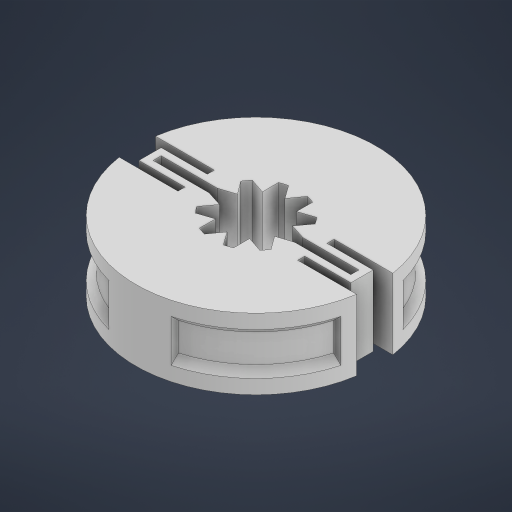
# Autodesk Inventor part: gear_grip
Saved by Autodesk Inventor 2024 (Build 280153000, 153)
## iProperties
Created: 2024-10-06
Part Number: gear_grip
Material: Generic
Document SubType Name: Modeling
Designer: loren
Density: 1 g/cm^3
Appearance: Default
Author: loren
## iProperties of the stored document gear-grip_3DPrint.ipt
Created: 2026-02-06
Part Number: gear-grip_3DPrint
Material: Generic
Document SubType Name: Modeling
Designer: lokies
Density: 1 g/cm^3
Appearance: Default
Author: lokies
Autodesk Inventor part; units mm, degrees
ref_plane "YZ Plane" through (0, 0, 0) normal (1, 0, 0) x (0, 1, 0)
ref_plane "XZ Plane" through (0, 0, 0) normal (0, 1, 0) x (-1, 0, 0)
ref_plane "XY Plane" through (0, 0, 0) normal (0, 0, 1) x (1, 0, 0)
sketch "Sketch1" plane through (0, 0, 0) normal (0, 0, 1) x (1, 0, 0)
  circle A0 centre (0, 0) radius 8.5
  dimension "d0" = 17
  constraints: 1 centre point, 1 coincident
  measures "d0" diameter of A0
extrude "Extrusion1" add sketch "Sketch1" along normal mid plane 5
sketch "Sketch2" plane through (0, 0, 2.5) normal (0, 0, 1) x (1, 0, 0)
  circle A0 centre (0, 0) radius 3.05
  dimension "d3" = 6.1
  constraints: 1 centre point, 1 coincident
  measures "d3" diameter of A0
extrude "Extrusion2" cut sketch "Sketch2" against normal through all
sketch "Sketch3" plane through (0, 0, 2.5) normal (0, 0, 1) x (1, 0, 0)
  circle A0 centre (0, 0) radius 3.05
  line L0 (-0.665337, 2.976546) -> (0, 2.05)
  line L1 (0, 2.05) -> (0.665337, 2.976546)
  line L2 (0, 2.05) -> (0, 3.05) construction
  dimension "d6" = 25.2
  dimension "d7" = 1
  constraints: 6 end point, 3 point on circle, 1 equal length, 1 horizontal alignment, 1 vertical
  measures "d7" distance of L0.end L2.end
extrude "Extrusion3" add sketch "Sketch3" against normal up to surface (5 mm away) contours L1 L0 A0 picked at (0.296238, 2.689452)
pattern_circular "Circular Pattern1" count 10 over 360 about axis through (0, 0, -10) along (0, 0, 1) of "Extrusion3"
chamfer "Chamfer1" distance 0.5 angle 45 33 edges at (-0.3327, -2.5133, -2.5) (0.3327, -2.5133, -2.5) (0.9425, -2.9007, -2.5) (-0.9425, -2.9007, -2.5) (1.2081, -2.2288, -2.5) (2.4675, -1.7927, -2.5) (1.7464, -1.8377, -2.5) (2.2875, -1.093, -2.5) (2.4931, 0.4603, -2.5) (2.2875, 1.093, -2.5) (2.4675, 1.7927, -2.5) (1.7464, 1.8377, -2.5) (1.2081, 2.2288, -2.5) (0.9425, 2.9007, -2.5) (0.3327, 2.5133, -2.5) (-0.3327, 2.5133, -2.5) (-0.9425, 2.9007, -2.5) (-1.2081, 2.2288, -2.5) (-1.7464, 1.8377, -2.5) (-2.4675, 1.7927, -2.5) (-2.2875, 1.093, -2.5) (-2.4931, 0.4603, -2.5) (-3.05, 0, -2.5) (-2.4931, -0.4603, -2.5) (-2.2875, -1.093, -2.5) (-2.4675, -1.7927, -2.5) (-1.7464, -1.8377, -2.5) (-1.2081, -2.2288, -2.5) (2.4931, -0.4603, -2.5) (3.0466, 0.1437, -2.5) (2.9007, 0.9425, -2.5) (2.9007, -0.9425, -2.5) (3.0466, -0.1437, -2.5)
sketch "Sketch5" plane through (0, 0, 2.5) normal (0, 0, 1) x (1, 0, 0)
  arc A0 (3.036464, -0.28703) -> (3.036464, 0.28703) centre (0, 0) ccw
  line L0 (3.036464, 0.28703) -> (7, 0.28703)
  line L1 (7, 0.28703) -> (7, -0.28703)
  line L2 (7, -0.28703) -> (3.036464, -0.28703)
  line L3 (3.036464, -0.28703) -> (3.036464, 0.28703)
  circle A1 centre (0, 0) radius 8.5
  line L4 (7.5, 0.78703) -> (4.236464, 0.78703)
  line L5 (4.236464, 0.78703) -> (4.236464, 1.28703)
  line L6 (4.236464, 1.28703) -> (8.401997, 1.28703)
  line L7 (7.5, -0.78703) -> (4.236464, -0.78703)
  line L8 (4.236464, -0.78703) -> (4.236464, -1.28703)
  line L9 (4.236464, -1.28703) -> (8.401997, -1.28703)
  line L10 (7.5, 0.78703) -> (7.5, -0.78703)
  point P0 (8.401997, -1.28703)
  point P1 (8.401997, 1.28703)
  dimension "d19" = 0.5
  dimension "d20" = 1.2
  dimension "d21" = 0.5
  dimension "d22" = 0.5
  dimension "d28" = 7
  dimension "d29" = 0.5
  constraints: 22 end point, 4 parallel, 3 horizontal, 3 perpendicular, 2 equal length, 2 point on circle, 1 vertical
  measures "d19" distance between parallel lines of L0 L4
  measures "d20" distance between parallel lines of L3 L5
  measures "d21" distance between parallel lines of L4 L6
  measures "d22" distance between parallel lines of L7 L2
  measures "d28" distance from line of point (0, 0) L1
  measures "d29" distance between parallel lines of L1 L10
extrude "Extrusion5" cut sketch "Sketch5" against normal through all contours L3 A0 | A0 L0 L1 L2 | A1 L9 L8 L7 L10 L4 L5 L6 picked at (6.71282, -1.120363)
pattern_circular "Circular Pattern2" count 2 over 360 about axis through (0, 0, -10) along (0, 0, 1) of "Extrusion5"
sketch "Sketch6" plane through (0, 0, 0) normal (0, 0, 1) x (1, 0, 0)
  arc A0 (7.691565, 2.199962) -> (2.199962, 7.691565) centre (0, 0) ccw
  line L0 (2.199962, 7.691565) -> (2.199962, 8.21037)
  arc A1 (8.401997, 1.28703) -> (-8.401997, 1.28703) centre (0, 0) ccw
  line L1 (7.691565, 2.199962) -> (8.21037, 2.199962)
  dimension "d30" = 60
  dimension "d31" = 0.5
  constraints: 4 end point, 4 point on circle, 1 centre point, 1 coincident, 1 horizontal, 1 perpendicular, 1 vertical
  measures "d31" radial gap between concentric circles of A1 A0
extrude "Extrusion6" cut sketch "Sketch6" along normal mid plane 3
chamfer "Chamfer2" distance 0.5 angle 45 2 edges at (5.6569, 5.6569, -1.5) (5.6569, 5.6569, 1.5)
pattern_circular "Circular Pattern3" count 4 over 360 about axis through (0, 0, -10) along (0, 0, 1) of "Extrusion6", "Chamfer2"
equation "\"d19\" = d18"
equation "\"d21\" = d19"
equation "\"d22\" = d19"
equation "\"d29\" = d19"
equation "\"d18\" = 0.5"
body "Solid1"
